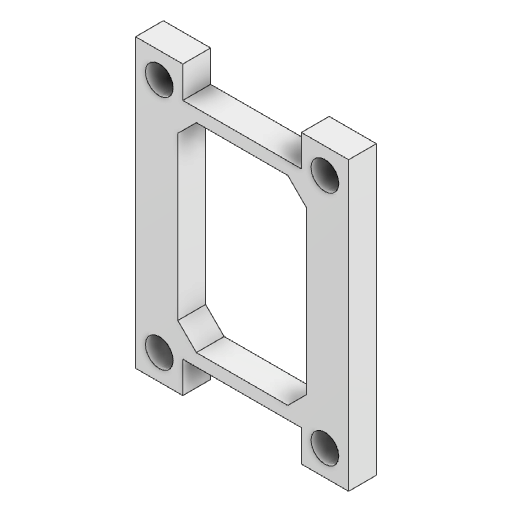
# Autodesk Inventor part: CFV4_Scale_HX711_Baseplate
Saved by Autodesk Inventor 2022 (Build 260153000, 153)
## iProperties
Created: 2022-07-20
Part Number: CFV4_Scale_HX711_Baseplate
Material: ABS-Kunststoff
Document SubType Name: Modeling
Designer: s-fau
Density: 1.06 g/cm^3
Appearance: Glatt - Weiß
Author: s-fau
Autodesk Inventor part; units mm, degrees
ref_plane "YZ Plane" through (0, 0, 0) normal (1, 0, 0) x (0, 1, 0)
ref_plane "XZ Plane" through (0, 0, 0) normal (0, 1, 0) x (-1, 0, 0)
ref_plane "XY Plane" through (0, 0, 0) normal (0, 0, 1) x (1, 0, 0)
sketch "Skizze1" plane through (0, 0, 0) normal (0, 0, 1) x (1, 0, 0)
  line L0 (0, 0) -> (23, 0)
  line L1 (23, 0) -> (23, -31)
  line L2 (23, -31) -> (0, -31)
  line L3 (0, -31) -> (0, 0)
  line L4 (2.56, -2.75) -> (20.44, -2.75) construction
  line L5 (20.44, -2.75) -> (20.44, -28.25) construction
  line L6 (20.44, -28.25) -> (2.56, -28.25) construction
  line L7 (2.56, -28.25) -> (2.56, -2.75) construction
  circle A0 centre (2.56, -2.75) radius 1.5
  circle A1 centre (20.44, -2.75) radius 1.5
  circle A2 centre (2.56, -28.25) radius 1.5
  circle A3 centre (20.44, -28.25) radius 1.5
  line L8 (4.56, -4.75) -> (18.44, -4.75)
  line L9 (18.44, -4.75) -> (18.44, -26.25)
  line L10 (18.44, -26.25) -> (4.56, -26.25)
  line L11 (4.56, -26.25) -> (4.56, -4.75)
  dimension "d0" = 23
  dimension "d1" = 31
  dimension "d2" = 17.88
  dimension "d3" = 25.5
  dimension "d4" = 2.75
  dimension "d5" = 2.56
  dimension "d6" = 3
  dimension "d7" = 3
  dimension "d8" = 3
  dimension "d9" = 3
  dimension "d10" = 2
  dimension "d11" = 2
  dimension "d12" = 2
  dimension "d13" = 2
  constraints: 24 end point, 6 parallel, 4 centre point, 4 coincident, 3 horizontal, 3 perpendicular
  measures "d0" distance of L1.end L2.end
  measures "d1" distance of L0.end L1.end
  measures "d2" distance of L4.start L4.end
  measures "d3" distance of L6.end L4.start
  measures "d4" distance between parallel lines of L0 L4
  measures "d5" distance between parallel lines of L1 L5
  measures "d6" diameter of A0
  measures "d7" diameter of A1
  measures "d8" diameter of A2
  measures "d9" diameter of A3
  measures "d10" distance between parallel lines of L7 L11
  measures "d11" distance between parallel lines of L4 L8
  measures "d12" distance between parallel lines of L5 L9
  measures "d13" distance between parallel lines of L6 L10
extrude "Extrusion1" add sketch "Skizze1" along normal blind 3
sketch "Skizze2" plane through (0, 0, 3) normal (0, 0, 1) x (1, 0, 0)
  line L0 (5.1, -31) -> (17.9, -31)
  line L1 (17.9, -31) -> (17.9, -27.6)
  line L2 (17.9, -27.6) -> (5.1, -27.6)
  line L3 (5.1, -27.6) -> (5.1, -31)
  line L4 (23, 0) -> (0, 0) projected
  line L5 (5.1, 0) -> (17.9, 0)
  line L6 (17.9, 0) -> (17.9, -3.4)
  line L7 (17.9, -3.4) -> (5.1, -3.4)
  line L8 (5.1, -3.4) -> (5.1, 0)
  line L9 (0, -31) -> (23, -31) projected
  line L10 (0, 0) -> (0, -31) projected
  dimension "d16" = 3.4
  dimension "d17" = 3.4
  dimension "d18" = 12.8
  dimension "d19" = 5.1
  constraints: 16 end point, 4 parallel, 3 collinear, 2 horizontal, 2 perpendicular, 1 point on line
  measures "d16" distance between parallel lines of L4 L7
  measures "d17" distance between parallel lines of L0 L2
  measures "d18" distance between parallel lines of L6 L8
  measures "d19" distance between parallel lines of L8 L10
extrude "Extrusion2" cut sketch "Skizze2" against normal blind 3
chamfer "Fase1" distance 2 angle 45 4 edges at (4.56, -4.75, 1.5) (18.44, -4.75, 1.5) (4.56, -26.25, 1.5) (18.44, -26.25, 1.5)
